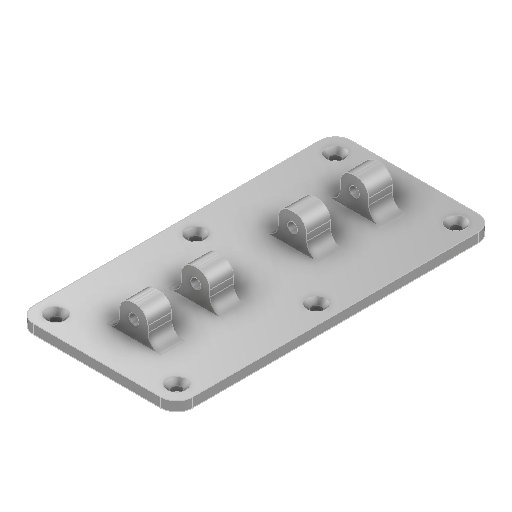
# Autodesk Inventor part: 3DP_PLA_Stand_Leg_Mount
Saved by Autodesk Inventor 2025 (Build 290162010, 162A)
## iProperties
Created: 2024-09-01
Part Number: 3DP_PLA_Stand_Leg_Mount
Material: Generic
Document SubType Name: Modeling
Designer: User
Density: 1 g/cm^3
Appearance: Rubber - Black - Version 1.1
Author: User
Autodesk Inventor part; units mm, degrees
ref_plane "YZ Plane" through (0, 0, 0) normal (1, 0, 0) x (0, 1, 0)
ref_plane "XZ Plane" through (0, 0, 0) normal (0, 1, 0) x (-1, 0, 0)
ref_plane "XY Plane" through (0, 0, 0) normal (0, 0, 1) x (1, 0, 0)
sketch "Sketch1" plane through (0, 0, 0) normal (0, 1, 0) x (-1, 0, 0)
  line L0 (25, 50) -> (-25, 50)
  line L1 (-25, 50) -> (-25, -50)
  line L2 (-25, -50) -> (25, -50)
  line L3 (25, -50) -> (25, 50)
  point P0 (0, 0)
  dimension "d0" = 100
  dimension "d1" = 50
  dimension "d2" = 25
  dimension "d3" = 50
  constraints: 8 end point, 2 parallel, 1 horizontal, 1 perpendicular
  measures "d0" distance of L0.end L1.end
  measures "d1" distance of L0.start L0.end
  measures "d2" distance from line of L3 point (0, 0)
  measures "d3" distance from line of L0 point (0, 0)
extrude "Extrusion1" add sketch "Sketch1" along normal blind 3
sketch "Sketch2" plane through (0, 3, 0) normal (0, 1, 0) x (1, 0, 0)
  line L0 (-4.5, -30.5) -> (4.5, -30.5)
  line L1 (4.5, -30.5) -> (4.5, -19.5)
  line L2 (4.5, -19.5) -> (-4.5, -19.5)
  line L3 (-4.5, -19.5) -> (-4.5, -30.5)
  line L4 (-4.5, -19.5) -> (-4.5, -19)
  line L5 (-4.5, -19) -> (4.5, -19)
  line L6 (4.5, -19) -> (4.5, -19.5)
  line L7 (-4.5, -19) -> (-4.5, -11.5)
  line L8 (-4.5, -11.5) -> (4.5, -11.5)
  line L9 (4.5, -11.5) -> (4.5, -19)
  line L10 (-4.5, -30.5) -> (-4.5, -31)
  line L11 (-4.5, -31) -> (4.5, -31)
  line L12 (4.5, -31) -> (4.5, -30.5)
  line L13 (-4.5, -31) -> (-4.5, -38.5)
  line L14 (-4.5, -38.5) -> (4.5, -38.5)
  line L15 (4.5, -38.5) -> (4.5, -31)
  line L16 (-25, -50) -> (25, -50) projected
  line L17 (31.6742, 0) -> (-41.419, 0)
  line L18 (-4.5, 30.5) -> (4.5, 30.5)
  line L19 (4.5, 30.5) -> (4.5, 19.5)
  line L20 (4.5, 19.5) -> (-4.5, 19.5)
  line L21 (-4.5, 19.5) -> (-4.5, 30.5)
  line L22 (-4.5, 19.5) -> (-4.5, 19)
  line L23 (-4.5, 19) -> (4.5, 19)
  line L24 (4.5, 19) -> (4.5, 19.5)
  line L25 (-4.5, 19) -> (-4.5, 11.5)
  line L26 (-4.5, 11.5) -> (4.5, 11.5)
  line L27 (4.5, 11.5) -> (4.5, 19)
  line L28 (-4.5, 30.5) -> (-4.5, 31)
  line L29 (-4.5, 31) -> (4.5, 31)
  line L30 (4.5, 31) -> (4.5, 30.5)
  line L31 (-4.5, 31) -> (-4.5, 38.5)
  line L32 (-4.5, 38.5) -> (4.5, 38.5)
  line L33 (4.5, 38.5) -> (4.5, 31)
  line L34 (-25, 50) -> (-25, -50) projected
  line L35 (25, -50) -> (25, 50) projected
  line L36 (25, 50) -> (-25, 50) projected
  point P0 (0, 0)
  point P1 (-19, -44)
  point P2 (-19, 0)
  point P3 (-19, 44)
  point P4 (19, -44)
  point P5 (19, 0)
  point P6 (19, 44)
  dimension "d6" = 9
  dimension "d7" = 11
  dimension "d8" = 4.5
  dimension "d9" = 0.5
  dimension "d10" = 0.5
  dimension "d11" = 27
  dimension "d12" = 7.5
  dimension "d14" = 11.5
  dimension "d27" = 6
  dimension "d28" = 6
  dimension "d29" = 6
  dimension "d30" = 6
  dimension "d31" = 50
  dimension "d43" = 39
  constraints: 66 end point, 14 point on line, 12 symmetric about line, 8 perpendicular, 4 vertical alignment, 3 horizontal alignment, 2 horizontal, 2 parallel, 1 collinear, 1 vertical
  measures "d6" distance between parallel lines of L1 L3
  measures "d7" distance between parallel lines of L0 L2
  measures "d8" distance from line of point (0, 0) L3
  measures "d9" distance between parallel lines of L11 L0
  measures "d10" distance between parallel lines of L2 L5
  measures "d11" distance between parallel lines of L8 L14
  measures "d12" distance between parallel lines of L14 L11
  measures "d14" distance between parallel lines of L16 L14
  measures "d27" distance from line of L34 point (-19, -44)
  measures "d28" distance from line of point (-19, -44) L16
  measures "d29" distance from line of L35 point (19, -44)
  measures "d30" distance from line of L36 point (19, 44)
  measures "d31" distance from line of L16 point (-19, 0)
  measures "d43" diameter of L2 L17
extrude "Extrusion2" add sketch "Sketch2" along normal blind 10 contours L11 L15 L14 L13 | L7 L8 L9 L5 | L31 L32 L33 L29 | L23 L27 L26 L25
sketch "Sketch3" plane through (-4.5, 3, 38.5) normal (0, 0, 1) x (1, 0, 0)
  line L0 (9, 0) -> (0, 0) projected
  line L1 (9, 0) -> (9, 10) projected
  line L2 (0, 10) -> (9, 10) projected
  line L3 (0, 0) -> (0, 10) projected
  point P0 (4.5, -3)
  point P1 (4.5, 5.5)
  point P2 (4.5, 10)
  dimension "d17" = 4.5
  dimension "d18" = 4.5
  constraints: 1 midpoint
  measures "d17" distance from line of L3 point (4.5, 5.5)
  measures "d18" distance of point (4.5, 10) point (4.5, 5.5)
hole "Hole1" at (0, 8.5, 38.5) direction (0, 0, -1) diameter 3.1 end through all
fillet "Fillet1" radius 4 16 edges at (-4.5, 13, 34.75) (4.5, 13, 34.75) (-4.5, 13, 15.25) (4.5, 13, 15.25) (-4.5, 13, -15.25) (4.5, 13, -15.25) (-4.5, 13, -34.75) (4.5, 13, -34.75) (-4.5, 3, -34.75) (-4.5, 3, -15.25) (-4.5, 3, 15.25) (-4.5, 3, 34.75) (4.5, 3, 34.75) (4.5, 3, 15.25) (4.5, 3, -15.25) (4.5, 3, -34.75)
hole "Hole2" at (-19, 3, 44) at (-19, 3, 0) at (-19, 3, -44) at (19, 3, 44) at (19, 3, 0) at (19, 3, -44) direction (0, -1, 0) diameter 3.1 end through all
chamfer "Chamfer1" distance 1.5 angle 45 6 edges at (19, 3, -45.55) (19, 3, -1.55) (-19, 3, -45.55) (19, 3, 42.45) (-19, 3, -1.55) (-19, 3, 42.45)
fillet "Fillet2" radius 5 4 edges at (25, 1.5, 50) (-25, 1.5, 50) (-25, 1.5, -50) (25, 1.5, -50)
equation "\"d2\" = 0.5 * d1"
equation "\"d3\" = 0.5 * d0"
equation "\"d8\" = 0.5 * d6"
equation "\"d10\" = d9"
equation "\"d12\" = -0.5 * d10 - 0.5 * d7 + 0.5 * d11 - 0.5 * d9"
equation "\"d28\" = d27"
equation "\"d29\" = d28"
equation "\"d30\" = d29"
equation "\"d18\" = d17"
body "Solid1"
